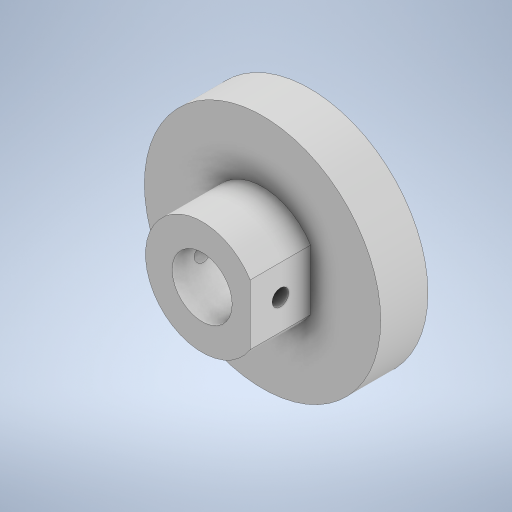
# Autodesk Inventor part: Project_Stationary_Wheel_Final
Saved by Autodesk Inventor 2024.3 (Build 283343000, 343)
## iProperties
Created: 2025-10-10
Part Number: Project_Stationary_Wheel_Final
Material: Generic
Document SubType Name: Sheet Metal
Designer: Rohith RN
Density: 1 g/cm^3
Sheet Metal Rule: Default_mm
Appearance: Default
Author: Rohith RN
Autodesk Inventor part; units mm, degrees
ref_plane "YZ Plane" through (0, 0, 0) normal (1, 0, 0) x (0, 1, 0)
ref_plane "XZ Plane" through (0, 0, 0) normal (0, 1, 0) x (-1, 0, 0)
ref_plane "XY Plane" through (0, 0, 0) normal (0, 0, 1) x (1, 0, 0)
sketch "Sketch1" plane through (0, 0, 0) normal (0, 0, 1) x (1, 0, 0)
  circle A0 centre (0, 0) radius 25
  dimension "d0" = 50
  constraints: 1 centre point, 1 coincident
  measures "d0" diameter of A0
extrude "Extrusion1" add sketch "Sketch1" along normal blind 10
sketch "Sketch14" plane through (0, 0, 10) normal (0, 0, 1) x (1, 0, 0)
  circle A0 centre (0, 0) radius 12
  line L0 (10.16, 0) -> (10.16, 6.3855)
  line L1 (10.16, -6.3855) -> (10.16, 0)
  dimension "d16" = 24
  constraints: 4 end point, 2 point on circle, 1 centre point, 1 coincident, 1 point on line, 1 vertical
  measures "d16" diameter of A0
extrude "Extrusion4" add sketch "Sketch14" along normal blind 12.771 contours L0 L1 A0 picked at (-4.553, 0)
sketch "Sketch19" plane through (0, 0, 22.771) normal (0, 0, 1) x (1, 0, 0)
  circle A0 centre (0, 0) radius 6.35
  dimension "d28" = 12.7
  constraints: 1 centre point, 1 coincident
  measures "d28" diameter of A0
extrude "Extrusion7" cut sketch "Sketch19" against normal blind 18
sketch "Sketch22" plane through (10.16, -6.3855, 10) normal (1, 0, 0) x (0, 0, -1)
  line L0 (-12.771, 0) -> (-12.771, 12.771) projected
  circle A0 centre (-6.3855, 6.3855) radius 1.75
  point P0 (10, 6.3855)
  dimension "d40" = 3.5
  constraints: 1 centre point
  measures "d40" diameter of A0
extrude "Extrusion10" cut sketch "Sketch22" against normal blind 25
sketch "Sketch23" plane through (0, 0, 4.771) normal (0, 0, 1) x (1, 0, 0)
  circle A0 centre (0, 0) radius 6.35
  dimension "d43" = 12.7
  constraints: 1 centre point, 1 coincident
  measures "d43" diameter of A0
extrude "Extrusion11" cut sketch "Sketch23" against normal blind 10
equation "\"BendRadius\" = Thickness"
equation "\"BendReliefWidth\" = Thickness"
equation "\"BendReliefDepth\" = 0.5 * Thickness"
equation "\"CornerReliefSize\" = 4 * Thickness"
equation "\"MinimumRemnant\" = 2 * Thickness"
equation "\"TransitionRadius\" = BendRadius"
equation "\"JacobiRadiusSize\" = BendRadius"
equation "\"GapSize\" = Thickness"
equation "\"Thickness\" = 0.5"
body "Solid1"
